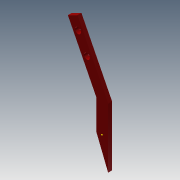
# Autodesk Inventor part: packa
Saved by Autodesk Inventor 2013 (Build 170138000, 138)
## iProperties
Created: 2013-02-02
Part Number: packa
Material: Generic
Document SubType Name: Modeling
Designer: idle-rug
Density: 1 g/cm^3
Author: idle-rug
Autodesk Inventor part; units mm, degrees
ref_plane "YZ Plane" through (0, 0, 0) normal (1, 0, 0) x (0, 1, 0)
ref_plane "XZ Plane" through (0, 0, 0) normal (0, 1, 0) x (-1, 0, 0)
ref_plane "XY Plane" through (0, 0, 0) normal (0, 0, 1) x (1, 0, 0)
sketch "Sketch1" plane through (0, 0, 0) normal (0, 1, 0) x (-1, 0, 0)
  line L0 (3, 15) -> (-3, 15)
  line L1 (-3, 15) -> (-3, -15)
  line L2 (3, 0) -> (-3, -15)
  line L3 (3, 0) -> (3, 15)
  line L4 (3, 15) -> (13, 34.9999)
  line L5 (-3, 15) -> (8, 37)
  line L6 (-3, 15) -> (0, 15)
  circle A0 centre (7.6833, 30.3666) radius 1.5
  circle A1 centre (12.1554, 39.3108) radius 1.5
  line L7 (8, 37) -> (12.4397, 45.8769)
  line L8 (13, 34.9999) -> (17.2387, 43.4774)
  line L9 (17.2387, 43.4774) -> (12.4397, 45.8769)
  point P0 (0, 0)
  constraints: 20 end point, 2 centre point, 2 parallel, 1 midpoint, 1 perpendicular
sketch "Sketch2" plane through (0, 0, 0) normal (0, 1, 0) x (-1, 0, 0)
  point P0 (0, 0)
extrude "Extrusion1" add sketch "Sketch1" along normal blind 2
body "Solid1"
